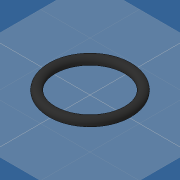
# Autodesk Inventor part: O-Ring_34x3.5
Saved by Autodesk Inventor 2019 (Build 230136000, 136)
## iProperties
Created: 2020-09-02
Part Number: O-Ring_34x3.5
Material: Generisch
Document SubType Name: Modeling
Designer: Stefan
Mass: 0.921883 g
Surface Area: 10.5358 cm^2
Volume: 0.921883 cm^3
Density: 1 g/cm^3
Appearance: Gummi - Schwarz
Author: Stefan
Autodesk Inventor part; units mm, degrees
ref_plane "YZ Plane" through (0, 0, 0) normal (1, 0, 0) x (0, 1, 0)
ref_plane "XZ Plane" through (0, 0, 0) normal (0, 1, 0) x (-1, 0, 0)
ref_plane "XY Plane" through (0, 0, 0) normal (0, 0, 1) x (1, 0, 0)
sketch "Skizze1" plane through (0, 0, 0) normal (0, 0, 1) x (1, 0, 0)
  circle A0 centre (-15.25, 0) radius 1.75
  line L0 (0, -2.45) -> (0, 2.45) projected
  point P0 (0, 0)
  dimension "d1" = 3.5
  dimension "d2" = 34
  constraints: 1 centre point, 1 horizontal alignment
  measures "d1" diameter of A0
revolve "Umdrehung1" add sketch "Skizze1" angle 360 about axis through (0, -10, 0) along (0, 1, 0)
